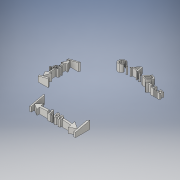
# Autodesk Inventor part: Team Pin Cad-Text
Saved by Autodesk Inventor 2016 (Build 200138000, 138)
## iProperties
Created: 2016-02-20
Part Number: Team Pin Cad-Text
Material: Generic
Document SubType Name: Modeling
Designer: RoksBot
Density: 1 g/cm^3
Appearance: White
Author: RoksBot
Autodesk Inventor part; units mm, degrees
ref_plane "YZ Plane" through (0, 0, 0) normal (1, 0, 0) x (0, 1, 0)
ref_plane "XZ Plane" through (0, 0, 0) normal (0, 1, 0) x (-1, 0, 0)
ref_plane "XY Plane" through (0, 0, 0) normal (0, 0, 1) x (1, 0, 0)
sketch "Sketch1" plane through (0, 0, 0) normal (0, 0, 1) x (1, 0, 0)
  line L0 (0, 0) -> (0, 8.6646) construction
  line L1 (20.9931, 1.27) -> (20.9931, 5.715)
  line L2 (20.9931, 5.715) -> (27.9781, 3.81)
  line L3 (27.9781, 3.81) -> (27.9781, 0)
  line L4 (27.9781, 0) -> (20.9931, 0)
  line L5 (20.9931, 1.27) -> (18.4531, 1.27)
  line L6 (18.4531, 1.27) -> (18.4531, 0)
  line L7 (18.4531, 0) -> (20.9931, 0)
  dimension "d0" = 20.9931
  dimension "d1" = 4.445
  dimension "d2" = 1.27
  dimension "d3" = 2.54
  dimension "d4" = 3.81
  dimension "d5" = 6.985
  constraints: 16 end point, 2 parallel, 2 perpendicular, 2 vertical, 1 horizontal, 1 horizontal alignment
  measures "d0" distance between parallel lines of L0 L1
  measures "d1" distance from line of L5 L1.end
  measures "d2" distance of L5.end L6.end
  measures "d3" distance between parallel lines of L1 L6
  measures "d4" distance of L2.end L3.end
  measures "d5" distance between parallel lines of L1 L3
revolve "Revolution1" add sketch "Sketch1" angle 360 about axis through (0, 0, 0) along (0, 1, 0)
sketch "Sketch2" plane through (0, 1.27, 0) normal (0, 1, 0) x (1, 0, 0)
  circle A0 centre (0, 0) radius 20.9931 projected
  circle A1 centre (0, 0) radius 27.9781 projected
  circle A2 centre (0, 0) radius 18.4531 projected
  line L0 (-4.2505, -7.1349) -> (4.1315, -7.1349) projected
  circle A3 centre (0, 0) radius 19.685 projected
  line L1 (-12.7595, -2.2222) -> (-12.7595, -29.7716) construction
  line L2 (12.6405, -2.2222) -> (12.6405, -30.8961) construction
  line L3 (-12.7549, -7.1349) -> (-31.6502, -7.1349) construction
  line L4 (0, 0) -> (17.3317, 30.0193) construction
  line L5 (-18.5066, 9.9103) -> (-25.4, 9.9103)
  line L6 (-18.9559, 9.0213) -> (-25.4, 9.0213)
  line L7 (-25.4, 9.0213) -> (-25.4, 9.9103)
  line L8 (-19.8985, -6.6904) -> (-25.4, -6.6904)
  line L9 (-25.4, -6.6904) -> (-25.4, -7.5794)
  line L10 (-25.4, -7.5794) -> (-19.5771, -7.5794)
  line L11 (0.1351, 9.4658) -> (-31.517, 9.4658) construction
  line L12 (-23.495, 9.0213) -> (-21.59, 5.7218)
  line L13 (-21.59, 5.7218) -> (-25.4, 5.7218)
  line L14 (-25.4, 5.7218) -> (-23.495, 9.0213)
  line L15 (-23.495, -6.6904) -> (-25.4, -3.3909)
  line L16 (-25.4, -3.3909) -> (-21.59, -3.3909)
  line L17 (-21.59, -3.3909) -> (-23.495, -6.6904)
  line L18 (-29.0818, 1.1654) -> (-16.5563, 1.1654) construction
  line L19 (-23.495, 6.8216) -> (-23.495, -4.4907) construction
  line L20 (-23.0505, 3.0704) -> (-23.9395, 3.0704)
  line L21 (-23.9395, 3.0704) -> (-23.9395, 5.7218)
  line L22 (-23.9395, 5.7218) -> (-23.0505, 5.7218)
  line L23 (-23.0505, 5.7218) -> (-23.0505, 3.0704)
  line L24 (-23.0505, 3.0704) -> (-23.9395, 5.7218) construction
  line L25 (-23.9395, 3.0704) -> (-23.0505, 5.7218) construction
  line L26 (-23.0505, -0.1046) -> (-23.9395, -0.1046)
  line L27 (-23.9395, -0.1046) -> (-23.9395, -3.3909)
  line L28 (-23.9395, -3.3909) -> (-23.0505, -3.3909)
  line L29 (-23.0505, -3.3909) -> (-23.0505, -0.1046)
  line L30 (-23.0505, -0.1046) -> (-23.9395, -3.3909) construction
  line L31 (-23.9395, -0.1046) -> (-23.0505, -3.3909) construction
  line L32 (-13.204, -16.3207) -> (-13.204, -24.5757)
  line L33 (-13.204, -24.5757) -> (-12.315, -24.5757)
  line L34 (-12.315, -24.5757) -> (-12.315, -17.0015)
  line L35 (12.196, -17.0871) -> (12.196, -24.5757)
  line L36 (12.196, -24.5757) -> (13.085, -24.5757)
  line L37 (13.085, -24.5757) -> (13.085, -16.4162)
  line L38 (-12.315, -22.6707) -> (-9.0154, -20.7657)
  line L39 (-9.0154, -20.7657) -> (-9.0154, -24.5757)
  line L40 (-9.0154, -24.5757) -> (-12.315, -22.6707)
  line L41 (12.196, -22.6707) -> (8.8965, -24.5757)
  line L42 (8.8965, -24.5757) -> (8.8965, -20.7657)
  line L43 (8.8965, -20.7657) -> (12.196, -22.6707)
  line L44 (-3.8695, -21.4007) -> (3.7505, -21.4007) construction
  line L45 (3.7505, -21.4007) -> (3.7505, -23.9407) construction
  line L46 (3.7505, -23.9407) -> (-3.8695, -23.9407) construction
  line L47 (-3.8695, -23.9407) -> (-3.8695, -21.4007) construction
  line L48 (-0.0595, -13.6296) -> (-0.0595, -32.797) construction
  line L49 (-9.0154, -22.6707) -> (8.8965, -22.6707) construction
  line L50 (-4.2505, -23.1152) -> (-9.0154, -23.1152)
  line L51 (-9.0154, -23.1152) -> (-9.0154, -22.2262)
  line L52 (-9.0154, -22.2262) -> (-4.2505, -22.2262)
  line L53 (-4.2505, -22.2262) -> (-4.2505, -23.1152)
  line L54 (-4.2505, -23.1152) -> (-9.0154, -22.2262) construction
  line L55 (-9.0154, -23.1152) -> (-4.2505, -22.2262) construction
  line L56 (4.1315, -22.2262) -> (8.8965, -22.2262)
  line L57 (8.8965, -22.2262) -> (8.8965, -23.1152)
  line L58 (8.8965, -23.1152) -> (4.1315, -23.1152)
  line L59 (4.1315, -23.1152) -> (4.1315, -22.2262)
  line L60 (4.1315, -22.2262) -> (8.8965, -23.1152) construction
  line L61 (8.8965, -22.2262) -> (4.1315, -23.1152) construction
  line L62 (10.1092, 18.3987) -> (11.0395, 20.0101)
  line L63 (11.0395, 20.0101) -> (11.8094, 19.5656)
  line L64 (11.8094, 19.5656) -> (10.8791, 17.9542)
  line L65 (12.9001, 20.8356) -> (18.6151, 20.8356) construction
  line L66 (18.6151, 20.8356) -> (18.6151, 18.2956) construction
  line L67 (18.6151, 18.2956) -> (12.9001, 18.2956) construction
  line L68 (12.9001, 18.2956) -> (12.9001, 20.8356) construction
  line L69 (11.0395, 20.0101) -> (12.9001, 20.0101)
  line L70 (12.9001, 20.0101) -> (12.9001, 19.1211)
  line L71 (12.9001, 19.1211) -> (11.0395, 19.1211)
  line L72 (11.0395, 19.1211) -> (11.0395, 20.0101)
  line L73 (11.0395, 20.0101) -> (12.9001, 19.1211) construction
  line L74 (12.9001, 20.0101) -> (11.0395, 19.1211) construction
  circle A4 centre (0, 0) radius 21.6281 construction
  line L75 (11.4654, -8.564) -> (6.3194, -8.564) projected
  spline S0 degree 2 poles (-5.588, 21.6946) (-5.7941, 21.1437) (-6.3523, 20.5845) (-6.8249, 20.4253) knots 0 0 0 1 2 2 2
  spline S1 degree 2 poles (-6.8249, 20.4253) (-7.6309, 20.1538) (-8.3698, 20.6637) knots 0 0 0 1 1 1
  spline S2 degree 2 poles (-8.3698, 20.6637) (-9.1257, 21.176) (-9.5009, 22.2898) knots 0 0 0 1 1 1
  spline S3 degree 2 poles (-9.5009, 22.2898) (-9.9155, 23.5209) (-9.5428, 24.3644) knots 0 0 0 1 1 1
  spline S4 degree 2 poles (-9.5428, 24.3644) (-9.2442, 25.0402) (-8.5628, 25.2697) knots 0 0 0 1 1 1
  spline S5 degree 2 poles (-8.5628, 25.2697) (-8.0315, 25.4487) (-7.6707, 25.3948) knots 0 0 0 1 1 1
  spline S6 degree 2 poles (-7.6707, 25.3948) (-7.2707, 25.3337) (-6.8857, 24.9779) knots 0 0 0 1 1 1
  spline S7 degree 2 poles (-6.8857, 24.9779) (-6.8036, 24.9036) (-6.7752, 24.8193) knots 0 0 0 1 1 1
  spline S8 degree 2 poles (-6.7752, 24.8193) (-6.7258, 24.6728) (-6.8778, 24.3972) (-7.0133, 24.3516) knots 0 0 0 1 2 2 2
  spline S9 degree 2 poles (-7.0133, 24.3516) (-7.2038, 24.2874) (-7.3829, 24.4556) knots 0 0 0 1 1 1
  spline S10 degree 2 poles (-7.3829, 24.4556) (-7.579, 24.6261) (-7.8224, 24.6461) knots 0 0 0 1 1 1
  spline S11 degree 2 poles (-7.8224, 24.6461) (-8.0095, 24.6688) (-8.3282, 24.5614) knots 0 0 0 1 1 1
  spline S12 degree 2 poles (-8.3282, 24.5614) (-8.7423, 24.4219) (-8.9034, 23.9556) knots 0 0 0 1 1 1
  spline S13 degree 2 poles (-8.9034, 23.9556) (-9.1045, 23.3902) (-8.8121, 22.5219) knots 0 0 0 1 1 1
  spline S14 degree 2 poles (-8.8121, 22.5219) (-8.543, 21.7231) (-7.5504, 20.9683) (-7.0521, 21.1361) knots 0 0 0 1 2 2 2
  spline S15 degree 2 poles (-7.0521, 21.1361) (-6.5135, 21.3175) (-6.2796, 21.9674) knots 0 0 0 1 1 1
  spline S16 degree 2 poles (-6.2796, 21.9674) (-6.219, 22.1266) (-6.0614, 22.1796) knots 0 0 0 1 1 1
  spline S17 degree 2 poles (-6.0614, 22.1796) (-5.9259, 22.2253) (-5.6259, 22.0857) (-5.5778, 21.9428) knots 0 0 0 1 2 2 2
  spline S18 degree 2 poles (-5.5778, 21.9428) (-5.5383, 21.8255) (-5.588, 21.6946) knots 0 0 0 1 1 1
  spline S19 degree 2 poles (-3.3163, 21.843) (-3.2858, 21.6561) (-3.501, 21.3664) (-3.6765, 21.3378) knots 0 0 0 1 2 2 2
  spline S20 degree 2 poles (-3.6765, 21.3378) (-3.8673, 21.3067) (-4.1513, 21.511) (-4.1824, 21.7018) knots 0 0 0 1 2 2 2
  spline S21 degree 2 poles (-4.1824, 21.7018) (-4.211, 21.8773) (-4.0079, 22.169) (-3.8171, 22.2001) knots 0 0 0 1 2 2 2
  spline S22 degree 2 poles (-3.8171, 22.2001) (-3.6416, 22.2287) (-3.3443, 22.0147) (-3.3163, 21.843) knots 0 0 0 1 2 2 2
  spline S23 degree 2 poles (2.1387, 22.0533) (2.1655, 21.9759) (2.1652, 21.9102) knots 0 0 0 1 1 1
  spline S24 degree 2 poles (2.1652, 21.9102) (2.1646, 21.7517) (1.9281, 21.5554) (1.785, 21.5559) knots 0 0 0 1 2 2 2
  spline S25 degree 2 poles (1.785, 21.5559) (1.5337, 21.5568) (1.4457, 21.7891) knots 0 0 0 1 1 1
  line L76 (1.4457, 21.7891) -> (1.1815, 22.4783)
  line L77 (1.1815, 22.4783) -> (-1.0647, 22.4866)
  line L78 (-1.0647, 22.4866) -> (-1.3301, 21.8033)
  spline S26 degree 2 poles (-1.3301, 21.8033) (-1.4199, 21.5678) (-1.6635, 21.5687) knots 0 0 0 1 1 1
  spline S27 degree 2 poles (-1.6635, 21.5687) (-1.8181, 21.5693) (-2.0455, 21.7712) (-2.0449, 21.9258) knots 0 0 0 1 2 2 2
  spline S28 degree 2 poles (-2.0449, 21.9258) (-2.0446, 21.9954) (-2.0212, 22.0572) knots 0 0 0 1 1 1
  line L79 (-2.0212, 22.0572) -> (-0.3813, 26.4043)
  spline S29 degree 2 poles (-0.3813, 26.4043) (-0.2759, 26.6822) (0.0411, 26.6811) knots 0 0 0 1 1 1
  spline S30 degree 2 poles (0.0411, 26.6811) (0.3659, 26.6799) (0.4539, 26.436) knots 0 0 0 1 1 1
  line L80 (0.4539, 26.436) -> (2.1387, 22.0533)
  line L81 (0.933, 23.2253) -> (0.0371, 25.5947)
  line L82 (0.0371, 25.5947) -> (-0.8145, 23.2318)
  line L83 (-0.8145, 23.2318) -> (0.933, 23.2253)
  spline S31 degree 2 poles (3.9548, 21.7365) (3.923, 21.5498) (3.6254, 21.3456) (3.4501, 21.3755) knots 0 0 0 1 2 2 2
  spline S32 degree 2 poles (3.4501, 21.3755) (3.2595, 21.4081) (3.0572, 21.6936) (3.0897, 21.8841) knots 0 0 0 1 2 2 2
  spline S33 degree 2 poles (3.0897, 21.8841) (3.1197, 22.0594) (3.4065, 22.2693) (3.597, 22.2368) knots 0 0 0 1 2 2 2
  spline S34 degree 2 poles (3.597, 22.2368) (3.7723, 22.2069) (3.9841, 21.908) (3.9548, 21.7365) knots 0 0 0 1 2 2 2
  spline S35 degree 2 poles (9.4674, 22.4288) (9.0295, 21.1444) (8.1193, 20.7032) knots 0 0 0 1 1 1
  spline S36 degree 2 poles (8.1193, 20.7032) (7.3833, 20.3415) (6.5856, 20.6135) knots 0 0 0 1 1 1
  line L84 (6.5856, 20.6135) -> (5.3085, 21.0489)
  line L85 (5.3085, 21.0489) -> (6.9218, 25.7803)
  line L86 (6.9218, 25.7803) -> (8.1952, 25.3461)
  spline S37 degree 2 poles (8.1952, 25.3461) (8.9819, 25.0778) (9.3756, 24.3636) knots 0 0 0 1 1 1
  spline S38 degree 2 poles (9.3756, 24.3636) (9.838, 23.5156) (9.4674, 22.4288) knots 0 0 0 1 1 1
  spline S39 degree 2 poles (8.7795, 22.6634) (9.0328, 23.4062) (8.7274, 23.9719) knots 0 0 0 1 1 1
  spline S40 degree 2 poles (8.7274, 23.9719) (8.4642, 24.4578) (7.9482, 24.6338) knots 0 0 0 1 1 1
  line L87 (7.9482, 24.6338) -> (7.3664, 24.8321)
  line L88 (7.3664, 24.8321) -> (6.2372, 21.5206)
  line L89 (6.2372, 21.5206) -> (6.8264, 21.3197)
  spline S41 degree 2 poles (6.8264, 21.3197) (7.3533, 21.14) (7.8144, 21.3423) knots 0 0 0 1 1 1
  spline S42 degree 2 poles (7.8144, 21.3423) (8.4638, 21.7376) (8.7795, 22.6634) knots 0 0 0 1 1 1
  line L90 (-26.1898, 0.2129) -> (-26.7929, 0.2129)
  line L91 (-26.7929, 0.2129) -> (-26.7929, 0.884)
  line L92 (-26.7929, 0.884) -> (-26.1898, 0.884)
  line L93 (-26.1898, 0.884) -> (-26.1898, 0.2129)
  spline S43 degree 2 poles (-23.8351, 1.0775) (-23.8351, 0.6761) (-24.3435, 0.1594) (-24.7881, 0.1594) knots 0 0 0 1 2 2 2
  spline S44 degree 2 poles (-24.7881, 0.1594) (-25.0104, 0.1594) (-25.3583, 0.287) (-25.4797, 0.4126) knots 0 0 0 1 2 2 2
  spline S45 degree 2 poles (-25.4797, 0.4126) (-25.6238, 0.5587) (-25.7782, 1.0219) (-25.7782, 1.345) knots 0 0 0 1 2 2 2
  spline S46 degree 2 poles (-25.7782, 1.345) (-25.7782, 1.6785) (-25.6341, 2.1972) (-25.4715, 2.3969) knots 0 0 0 1 2 2 2
  spline S47 degree 2 poles (-25.4715, 2.3969) (-25.3171, 2.5862) (-24.8149, 2.8003) (-24.4711, 2.8003) knots 0 0 0 1 2 2 2
  spline S48 degree 2 poles (-24.4711, 2.8003) (-24.3455, 2.8003) (-24.0944, 2.7674) (-24.0491, 2.7571) knots 0 0 0 1 2 2 2
  line L94 (-24.0491, 2.7571) -> (-24.0491, 2.2589)
  line L95 (-24.0491, 2.2589) -> (-24.0944, 2.2589)
  spline S49 degree 2 poles (-24.0944, 2.2589) (-24.1397, 2.2816) (-24.3455, 2.3372) (-24.4773, 2.3372) knots 0 0 0 1 2 2 2
  spline S50 degree 2 poles (-24.4773, 2.3372) (-24.7757, 2.3372) (-25.101, 2.0222) (-25.1401, 1.7299) knots 0 0 0 1 2 2 2
  spline S51 degree 2 poles (-25.1401, 1.7299) (-25.0145, 1.8102) (-24.7572, 1.9049) (-24.5946, 1.9049) knots 0 0 0 1 2 2 2
  spline S52 degree 2 poles (-24.5946, 1.9049) (-24.4567, 1.9049) (-24.2159, 1.8308) (-24.1232, 1.7608) knots 0 0 0 1 2 2 2
  spline S53 degree 2 poles (-24.1232, 1.7608) (-23.9915, 1.66) (-23.8351, 1.3327) (-23.8351, 1.0775) knots 0 0 0 1 2 2 2
  spline S54 degree 2 poles (-24.5781, 0.6946) (-24.5287, 0.7564) (-24.4752, 0.9004) (-24.4752, 1.0466) knots 0 0 0 1 2 2 2
  spline S55 degree 2 poles (-24.4752, 1.0466) (-24.4752, 1.1701) (-24.537, 1.3306) (-24.5925, 1.378) knots 0 0 0 1 2 2 2
  spline S56 degree 2 poles (-24.5925, 1.378) (-24.6502, 1.4274) (-24.7922, 1.4624) (-24.8725, 1.4624) knots 0 0 0 1 2 2 2
  spline S57 degree 2 poles (-24.8725, 1.4624) (-24.9404, 1.4624) (-25.0804, 1.4274) (-25.1421, 1.4027) knots 0 0 0 1 2 2 2
  spline S58 degree 2 poles (-25.1421, 1.4027) (-25.1421, 1.3862) (-25.1462, 1.308) (-25.1462, 1.2483) knots 0 0 0 1 2 2 2
  spline S59 degree 2 poles (-25.1462, 1.2483) (-25.1462, 1.0281) (-25.0701, 0.7625) (-25.0104, 0.6946) knots 0 0 0 1 2 2 2
  spline S60 degree 2 poles (-25.0104, 0.6946) (-24.9672, 0.639) (-24.8519, 0.5917) (-24.7902, 0.5917) knots 0 0 0 1 2 2 2
  spline S61 degree 2 poles (-24.7902, 0.5917) (-24.7387, 0.5917) (-24.6193, 0.6431) (-24.5781, 0.6946) knots 0 0 0 1 2 2 2
  spline S62 degree 2 poles (-21.6532, 1.0733) (-21.6532, 0.8737) (-21.7891, 0.5361) (-21.9229, 0.4147) knots 0 0 0 1 2 2 2
  spline S63 degree 2 poles (-21.9229, 0.4147) (-22.0567, 0.2932) (-22.4231, 0.1594) (-22.6906, 0.1594) knots 0 0 0 1 2 2 2
  spline S64 degree 2 poles (-22.6906, 0.1594) (-22.9747, 0.1615) (-23.3822, 0.2541) (-23.516, 0.3138) knots 0 0 0 1 2 2 2
  line L96 (-23.516, 0.3138) -> (-23.516, 0.8675)
  line L97 (-23.516, 0.8675) -> (-23.4584, 0.8675)
  spline S65 degree 2 poles (-23.4584, 0.8675) (-23.409, 0.8407) (-23.2896, 0.7708) (-23.1929, 0.7337) knots 0 0 0 1 2 2 2
  spline S66 degree 2 poles (-23.1929, 0.7337) (-23.1023, 0.6987) (-22.915, 0.6514) (-22.8018, 0.6514) knots 0 0 0 1 2 2 2
  spline S67 degree 2 poles (-22.8018, 0.6514) (-22.703, 0.6514) (-22.4725, 0.7008) (-22.4025, 0.7666) knots 0 0 0 1 2 2 2
  spline S68 degree 2 poles (-22.4025, 0.7666) (-22.351, 0.8181) (-22.2934, 0.9437) (-22.2934, 1.0486) knots 0 0 0 1 2 2 2
  spline S69 degree 2 poles (-22.2934, 1.0486) (-22.2934, 1.1392) (-22.3675, 1.2668) (-22.4272, 1.3059) knots 0 0 0 1 2 2 2
  spline S70 degree 2 poles (-22.4272, 1.3059) (-22.5136, 1.3636) (-22.7606, 1.3965) (-22.8491, 1.3965) knots 0 0 0 1 2 2 2
  spline S71 degree 2 poles (-22.8491, 1.3965) (-22.9891, 1.3965) (-23.2546, 1.3512) (-23.3514, 1.3265) knots 0 0 0 1 2 2 2
  line L98 (-23.3514, 1.3265) -> (-23.4069, 1.3265)
  line L99 (-23.4069, 1.3265) -> (-23.4069, 2.7529)
  line L100 (-23.4069, 2.7529) -> (-21.7232, 2.7529)
  line L101 (-21.7232, 2.7529) -> (-21.7232, 2.2734)
  line L102 (-21.7232, 2.2734) -> (-22.8038, 2.2734)
  line L103 (-22.8038, 2.2734) -> (-22.8038, 1.8514)
  spline S72 degree 2 poles (-22.8038, 1.8514) (-22.7524, 1.8555) (-22.6104, 1.8596) (-22.5713, 1.8596) knots 0 0 0 1 2 2 2
  spline S73 degree 2 poles (-22.5713, 1.8596) (-22.3881, 1.8596) (-22.0793, 1.7855) (-21.9579, 1.7094) knots 0 0 0 1 2 2 2
  spline S74 degree 2 poles (-21.9579, 1.7094) (-21.8138, 1.6147) (-21.6532, 1.2998) (-21.6532, 1.0733) knots 0 0 0 1 2 2 2
  line L104 (-1.9315, -23.9397) -> (-3.6091, -23.9397)
  line L105 (-3.6091, -23.9397) -> (-3.6091, -23.4971)
  line L106 (-3.6091, -23.4971) -> (-3.0739, -23.4971)
  line L107 (-3.0739, -23.4971) -> (-3.0739, -22.153)
  line L108 (-3.0739, -22.153) -> (-3.6091, -22.153)
  line L109 (-3.6091, -22.153) -> (-3.6091, -21.7393)
  spline S75 degree 2 poles (-3.6091, -21.7393) (-3.4918, -21.7393) (-3.2592, -21.7084) (-3.1892, -21.6755) knots 0 0 0 1 2 2 2
  spline S76 degree 2 poles (-3.1892, -21.6755) (-3.1089, -21.6343) (-3.0184, -21.4964) (-3.0101, -21.3935) knots 0 0 0 1 2 2 2
  line L110 (-3.0101, -21.3935) -> (-2.4544, -21.3935)
  line L111 (-2.4544, -21.3935) -> (-2.4544, -23.4971)
  line L112 (-2.4544, -23.4971) -> (-1.9315, -23.4971)
  line L113 (-1.9315, -23.4971) -> (-1.9315, -23.9397)
  line L114 (-0.8715, -23.9397) -> (-1.4746, -23.9397)
  line L115 (-1.4746, -23.9397) -> (-1.4746, -23.2686)
  line L116 (-1.4746, -23.2686) -> (-0.8715, -23.2686)
  line L117 (-0.8715, -23.2686) -> (-0.8715, -23.9397)
  spline S77 degree 2 poles (1.4647, -22.6697) (1.4647, -22.999) (1.3597, -23.493) (1.2424, -23.6597) knots 0 0 0 1 2 2 2
  spline S78 degree 2 poles (1.2424, -23.6597) (1.1272, -23.8244) (0.7546, -23.9932) (0.487, -23.9932) knots 0 0 0 1 2 2 2
  spline S79 degree 2 poles (0.487, -23.9932) (0.2174, -23.9932) (-0.1531, -23.8244) (-0.2705, -23.6556) knots 0 0 0 1 2 2 2
  spline S80 degree 2 poles (-0.2705, -23.6556) (-0.3878, -23.4889) (-0.4928, -22.999) (-0.4928, -22.6697) knots 0 0 0 1 2 2 2
  spline S81 degree 2 poles (-0.4928, -22.6697) (-0.4928, -22.3321) (-0.3878, -21.8546) (-0.2684, -21.6817) knots 0 0 0 1 2 2 2
  spline S82 degree 2 poles (-0.2684, -21.6817) (-0.149, -21.5129) (0.2277, -21.3482) (0.487, -21.3482) knots 0 0 0 1 2 2 2
  spline S83 degree 2 poles (0.487, -21.3482) (0.7608, -21.3482) (1.1272, -21.5211) (1.2445, -21.692) knots 0 0 0 1 2 2 2
  spline S84 degree 2 poles (1.2445, -21.692) (1.3597, -21.8587) (1.4647, -22.3506) (1.4647, -22.6697) knots 0 0 0 1 2 2 2
  spline S85 degree 2 poles (0.8246, -22.6697) (0.8246, -22.1983) (0.6702, -21.8175) (0.487, -21.8175) knots 0 0 0 1 2 2 2
  spline S86 degree 2 poles (0.487, -21.8175) (0.3038, -21.8175) (0.1474, -22.1983) (0.1474, -22.6717) knots 0 0 0 1 2 2 2
  spline S87 degree 2 poles (0.1474, -22.6717) (0.1474, -23.1369) (0.3038, -23.5239) (0.487, -23.5239) knots 0 0 0 1 2 2 2
  spline S88 degree 2 poles (0.487, -23.5239) (0.6681, -23.5239) (0.8246, -23.1369) (0.8246, -22.6697) knots 0 0 0 1 2 2 2
  spline S89 degree 2 poles (3.6898, -22.6697) (3.6898, -22.999) (3.5848, -23.493) (3.4675, -23.6597) knots 0 0 0 1 2 2 2
  spline S90 degree 2 poles (3.4675, -23.6597) (3.3522, -23.8244) (2.9797, -23.9932) (2.7121, -23.9932) knots 0 0 0 1 2 2 2
  spline S91 degree 2 poles (2.7121, -23.9932) (2.4424, -23.9932) (2.0719, -23.8244) (1.9546, -23.6556) knots 0 0 0 1 2 2 2
  spline S92 degree 2 poles (1.9546, -23.6556) (1.8373, -23.4889) (1.7323, -22.999) (1.7323, -22.6697) knots 0 0 0 1 2 2 2
  spline S93 degree 2 poles (1.7323, -22.6697) (1.7323, -22.3321) (1.8373, -21.8546) (1.9567, -21.6817) knots 0 0 0 1 2 2 2
  spline S94 degree 2 poles (1.9567, -21.6817) (2.0761, -21.5129) (2.4527, -21.3482) (2.7121, -21.3482) knots 0 0 0 1 2 2 2
  spline S95 degree 2 poles (2.7121, -21.3482) (2.9858, -21.3482) (3.3522, -21.5211) (3.4696, -21.692) knots 0 0 0 1 2 2 2
  spline S96 degree 2 poles (3.4696, -21.692) (3.5848, -21.8587) (3.6898, -22.3506) (3.6898, -22.6697) knots 0 0 0 1 2 2 2
  spline S97 degree 2 poles (3.0497, -22.6697) (3.0497, -22.1983) (2.8953, -21.8175) (2.7121, -21.8175) knots 0 0 0 1 2 2 2
  spline S98 degree 2 poles (2.7121, -21.8175) (2.5289, -21.8175) (2.3725, -22.1983) (2.3725, -22.6717) knots 0 0 0 1 2 2 2
  spline S99 degree 2 poles (2.3725, -22.6717) (2.3725, -23.1369) (2.5289, -23.5239) (2.7121, -23.5239) knots 0 0 0 1 2 2 2
  spline S100 degree 2 poles (2.7121, -23.5239) (2.8932, -23.5239) (3.0497, -23.1369) (3.0497, -22.6697) knots 0 0 0 1 2 2 2
  line L118 (14.9981, 18.3192) -> (13.3206, 18.3192)
  line L119 (13.3206, 18.3192) -> (13.3206, 18.7618)
  line L120 (13.3206, 18.7618) -> (13.8557, 18.7618)
  line L121 (13.8557, 18.7618) -> (13.8557, 20.1059)
  line L122 (13.8557, 20.1059) -> (13.3206, 20.1059)
  line L123 (13.3206, 20.1059) -> (13.3206, 20.5196)
  spline S101 degree 2 poles (13.3206, 20.5196) (13.4379, 20.5196) (13.6705, 20.5505) (13.7405, 20.5834) knots 0 0 0 1 2 2 2
  spline S102 degree 2 poles (13.7405, 20.5834) (13.8207, 20.6246) (13.9113, 20.7625) (13.9195, 20.8654) knots 0 0 0 1 2 2 2
  line L124 (13.9195, 20.8654) -> (14.4753, 20.8654)
  line L125 (14.4753, 20.8654) -> (14.4753, 18.7618)
  line L126 (14.4753, 18.7618) -> (14.9981, 18.7618)
  line L127 (14.9981, 18.7618) -> (14.9981, 18.3192)
  line L128 (16.0582, 18.3192) -> (15.4551, 18.3192)
  line L129 (15.4551, 18.3192) -> (15.4551, 18.9902)
  line L130 (15.4551, 18.9902) -> (16.0582, 18.9902)
  line L131 (16.0582, 18.9902) -> (16.0582, 18.3192)
  spline S103 degree 2 poles (18.3697, 19.1796) (18.3697, 18.98) (18.2338, 18.6424) (18.1, 18.5209) knots 0 0 0 1 2 2 2
  spline S104 degree 2 poles (18.1, 18.5209) (17.9662, 18.3995) (17.5999, 18.2657) (17.3323, 18.2657) knots 0 0 0 1 2 2 2
  spline S105 degree 2 poles (17.3323, 18.2657) (17.0482, 18.2678) (16.6407, 18.3604) (16.5069, 18.4201) knots 0 0 0 1 2 2 2
  line L132 (16.5069, 18.4201) -> (16.5069, 18.9738)
  line L133 (16.5069, 18.9738) -> (16.5645, 18.9738)
  spline S106 degree 2 poles (16.5645, 18.9738) (16.6139, 18.947) (16.7333, 18.877) (16.83, 18.84) knots 0 0 0 1 2 2 2
  spline S107 degree 2 poles (16.83, 18.84) (16.9206, 18.805) (17.1079, 18.7577) (17.2211, 18.7577) knots 0 0 0 1 2 2 2
  spline S108 degree 2 poles (17.2211, 18.7577) (17.3199, 18.7577) (17.5505, 18.8071) (17.6204, 18.8729) knots 0 0 0 1 2 2 2
  spline S109 degree 2 poles (17.6204, 18.8729) (17.6719, 18.9244) (17.7295, 19.0499) (17.7295, 19.1549) knots 0 0 0 1 2 2 2
  spline S110 degree 2 poles (17.7295, 19.1549) (17.7295, 19.2455) (17.6554, 19.3731) (17.5957, 19.4122) knots 0 0 0 1 2 2 2
  spline S111 degree 2 poles (17.5957, 19.4122) (17.5093, 19.4698) (17.2623, 19.5028) (17.1738, 19.5028) knots 0 0 0 1 2 2 2
  spline S112 degree 2 poles (17.1738, 19.5028) (17.0338, 19.5028) (16.7683, 19.4575) (16.6715, 19.4328) knots 0 0 0 1 2 2 2
  line L134 (16.6715, 19.4328) -> (16.616, 19.4328)
  line L135 (16.616, 19.4328) -> (16.616, 20.8592)
  line L136 (16.616, 20.8592) -> (18.2997, 20.8592)
  line L137 (18.2997, 20.8592) -> (18.2997, 20.3796)
  line L138 (18.2997, 20.3796) -> (17.2191, 20.3796)
  line L139 (17.2191, 20.3796) -> (17.2191, 19.9577)
  spline S113 degree 2 poles (17.2191, 19.9577) (17.2705, 19.9618) (17.4125, 19.9659) (17.4517, 19.9659) knots 0 0 0 1 2 2 2
  spline S114 degree 2 poles (17.4517, 19.9659) (17.6349, 19.9659) (17.9436, 19.8918) (18.065, 19.8156) knots 0 0 0 1 2 2 2
  spline S115 degree 2 poles (18.065, 19.8156) (18.2091, 19.721) (18.3697, 19.406) (18.3697, 19.1796) knots 0 0 0 1 2 2 2
  point P0 (-10.4828, 14.7667)
  point P1 (-23.495, 4.3961)
  point P2 (-23.495, -1.7477)
  point P3 (-10.1153, -22.6707)
  point P4 (9.9963, -22.6707)
  point P5 (-3.8695, -22.6707)
  point P6 (-0.0595, -23.9407)
  point P7 (-6.633, -22.6707)
  point P8 (6.514, -22.6707)
  point P9 (11.9698, 19.5656)
  point P10 (11.9698, 19.5656)
  point P11 (18.6151, 19.5656)
  dimension "d7" = 39.37
  dimension "d9" = 25.4
  dimension "d11" = 0.889
  dimension "d13" = 25.4
  dimension "d14" = 0.889
  dimension "d15" = 0.4445
  dimension "d16" = 16.6007
  dimension "d17" = 0.4445
  dimension "d18" = 3.81
  dimension "d19" = 1.905
  dimension "d20" = 1.27
  dimension "d21" = 0.889
  dimension "d22" = 0.4445
  dimension "d23" = 8.255
  dimension "d24" = 0.4445
  dimension "d25" = 3.81
  dimension "d26" = 7.62
  dimension "d27" = 2.54
  dimension "d28" = 0.889
  dimension "d29" = 0.381
  dimension "d30" = 0.381
  dimension "d31" = 0.889
  dimension "d32" = 0.4445
  dimension "d33" = 5.715
  dimension "d34" = 2.54
  dimension "d35" = 27.94
  dimension "d36" = 0.889
  dimension "d38" = 60
  dimension "d39" = 0.635
  constraints: 132 end point, 16 midpoint, 16 point on line, 14 perpendicular, 13 horizontal, 12 parallel, 8 vertical, 5 equal length, 5 horizontal alignment, 3 vertical alignment, 1 centre point, 1 coincident, 1 collinear, 50 other
  measures "d7" diameter of A3
  measures "d9" distance between parallel lines of L2 L1
  measures "d11" distance between parallel lines of L6 L5
  measures "d13" horizontal distance of A1.centre L5.end
  measures "d14" distance between parallel lines of L10 L8
  measures "d15" distance between parallel lines of L10 L3
  measures "d16" distance from line of L11.start L0
  measures "d17" distance between parallel lines of L11 L5
  measures "d18" distance of L12.end L13.end
  measures "d19" distance between parallel lines of L18 L20
  measures "d20" distance between parallel lines of L18 L26
  measures "d21" distance of L32.end L33.end
  measures "d22" distance between parallel lines of L1 L32
  measures "d23" distance of L32.start L32.end
  measures "d24" distance between parallel lines of L2 L35
  measures "d25" distance of L38.end L39.end
  measures "d26" distance of L45.end L46.end
  measures "d27" distance of L44.end L45.end
  measures "d28" distance of L52.end L50.start
  measures "d29" distance between parallel lines of L47 L53
  measures "d30" distance between parallel lines of L45 L59
  measures "d31" distance of L62.end L63.end
  measures "d32" distance between parallel lines of L4 L62
  measures "d33" distance of L65.start L65.end
  measures "d34" distance of L65.end L66.end
  measures "d35" distance of A1.centre L65.end
  measures "d36" distance of L69.end L70.end
  measures "d38" angle of L0 L4
extrude "Extrusion1" cut sketch "Sketch2" along normal through all contours L41 L42 L43 | L38 L39 L40 | L15 L16 L17 | L12 L13 L14 | A0 L62 L72 L71 L64 | L37 L36 L35 A0 | L71 L72 L63 L64 | L64 L63 L69 L70 L71 | A0 L6 L7 L5 | L34 L33 L32 A0 | A0 L10 L9 L8 | L58 L59 L56 L42 | L52 L53 L50 L39 | L23 L20 L21 L13 | L27 L26 L29 L16 | S0 S1 S2 S3 S4 S5 S6 S7 S8 S9 S10 S11 S12 S13 S14 S15 S16 S17 S18 | S19 S20 S21 S22 | S23 S24 S25 L76 L77 L78 S26 S27 S28 L79 S29 S30 L80 | S31 S32 S33 S34 | S35 S36 L84 L85 L86 S37 S38 | L90 L91 L92 L93 | S43 S44 S45 S46 S47 S48 L94 L95 S49 S50 S51 S52 S53 | S62 S63 S64 L96 L97 S65 S66 S67 S68 S69 S70 S71 L98 L99 L100 L101 L102 L103 S72 S73 S74 | L104 L105 L106 L107 L108 L109 S75 S76 L110 L111 L112 L113 | L114 L115 L116 L117 | S77 S78 S79 S80 S81 S82 S83 S84 | S89 S90 S91 S92 S93 S94 S95 S96 | L118 L119 L120 L121 L122 L123 S101 S102 L124 L125 L126 L127 | L128 L129 L130 L131 | S103 S104 S105 L132 L133 S106 S107 S108 S109 S110 S111 S112 L134 L135 L136 L137 L138 L139 S113 S114 S115 keep common part
sketch "Sketch3" plane through (-25.4, 1.27, -9.9103) normal (0, 1, 0) x (1, 0, 0)
  circle A0 centre (25.4, -9.7833) radius 18.415 projected
  circle A1 centre (25.4, -9.7833) radius 19.685 projected
  circle A2 centre (25.4, -9.9103) radius 27.9781 projected
  line L0 (48.2883, -22.4902) -> (51.5753, -10.223)
  line L1 (51.5753, -10.223) -> (50.3486, -9.8943)
  line L2 (50.3486, -9.8943) -> (47.0616, -22.1615)
  line L3 (47.0616, -22.1615) -> (48.2883, -22.4902)
  line L4 (48.2883, -22.4902) -> (50.3486, -9.8943) construction
  line L5 (51.5753, -10.223) -> (47.0616, -22.1615) construction
  line L6 (48.9988, -13.214) -> (48.1771, -16.2809)
  line L7 (48.1771, -16.2809) -> (50.2625, -16.8396)
  line L8 (50.2625, -16.8396) -> (51.0843, -13.7728)
  line L9 (51.0843, -13.7728) -> (48.9988, -13.214)
  line L10 (48.9988, -13.214) -> (50.2625, -16.8396) construction
  line L11 (48.1771, -16.2809) -> (51.0843, -13.7728) construction
  line L12 (50.3486, -9.8943) -> (47.0188, -10.0539)
  line L13 (47.0188, -10.0539) -> (50.0856, -10.8756)
  line L14 (48.9988, -13.214) -> (46.3614, -12.5073)
  line L15 (46.3614, -12.5073) -> (48.7359, -14.1954)
  line L16 (51.3123, -11.2043) -> (52.2937, -11.4673)
  line L17 (52.2937, -11.4673) -> (51.148, -11.8177)
  line L18 (25.4, -9.9103) -> (37.7185, -9.9103) construction
  line L19 (51.0843, -13.7728) -> (51.6363, -13.9207)
  line L20 (51.6363, -13.9207) -> (50.8193, -13.0444)
  line L21 (50.8193, -13.0444) -> (50.6549, -13.6578) construction
  point P0 (49.3184, -16.1922)
  point P1 (49.6307, -15.0268)
  dimension "d42" = 3.175
  dimension "d43" = 3.175
  dimension "d44" = 1.016
  dimension "d45" = 1.27
  dimension "d46" = 1.016
  dimension "d47" = 1.016
  dimension "d49" = 0.635
  dimension "d50" = 3.175
  dimension "d51" = 12.7
  dimension "d52" = 2.159
  dimension "d53" = 2.54
  dimension "d54" = 24.765
  dimension "d55" = 0.635
  dimension "d56" = 24.9488
  dimension "d57" = 24.9488
  dimension "d58" = 15
  dimension "d59" = 1.016
  dimension "d60" = 0.635
  constraints: 44 end point, 10 point on line, 6 parallel, 4 midpoint, 3 perpendicular, 1 horizontal
  measures "d42" distance from line of L2 L12.end
  measures "d43" distance from line of L2 L14.end
  measures "d44" distance of L6.start L15.end
  measures "d45" distance between parallel lines of L0 L2
  measures "d46" distance of L1.end L13.end
  measures "d47" distance of L16.start L16.end
  measures "d49" distance of L16.start L17.end
  measures "d50" distance of L7.end L8.end
  measures "d51" distance between parallel lines of L3 L1
  measures "d52" distance between parallel lines of L8 L6
  measures "d53" distance between parallel lines of L14 L13
  measures "d54" distance of point (25.4, -9.91) point (49.631, -15.027)
  measures "d55" distance from line of L0 point (49.631, -15.027)
  measures "d56" distance of A0.centre L1.end
  measures "d57" distance of A0.centre L2.end
  measures "d58" angle of L9 L18
  measures "d59" distance from line of L0 L19.end
  measures "d60" distance from line of L9 L20.end
extrude "Extrusion2" [suppressed]
equation "\"d15\" = 0.5 * d14"
equation "\"d17\" = 0.5 * d11"
equation "\"d22\" = 0.5 * d21"
equation "\"d24\" = d22"
equation "\"d32\" = 0.5 * d31"
body "Solid1"
